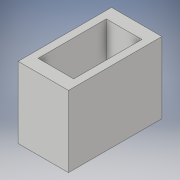
# Autodesk Inventor part: COXA_B
Saved by Autodesk Inventor 2017 (Build 210142000, 142)
## iProperties
Created: 2017-09-18
Part Number: COXA_B
Material: Generic
Document SubType Name: Modeling
Designer: Alexander Miller
Density: 1 g/cm^3
Appearance: Default
Author: Alexander Miller
Autodesk Inventor part; units mm, degrees
ref_plane "YZ Plane" through (0, 0, 0) normal (1, 0, 0) x (0, 1, 0)
ref_plane "XZ Plane" through (0, 0, 0) normal (0, 1, 0) x (-1, 0, 0)
ref_plane "XY Plane" through (0, 0, 0) normal (0, 0, 1) x (1, 0, 0)
sketch "Sketch1" plane through (0, 0, 0) normal (0, 1, 0) x (-1, 0, 0)
  line L0 (8.5, 15.75) -> (-8.5, 15.75)
  line L1 (-8.5, 15.75) -> (-8.5, -15.75)
  line L2 (-8.5, -15.75) -> (8.5, -15.75)
  line L3 (8.5, -15.75) -> (8.5, 15.75)
  point P0 (0, 0)
  point P1 (0, -15.75)
  point P2 (8.5, 0)
  dimension "d0" = 17
  dimension "d1" = 31.5
  constraints: 8 end point, 2 midpoint, 2 parallel, 1 horizontal, 1 horizontal alignment, 1 perpendicular, 1 vertical alignment
  measures "d0" distance of L1.end L2.end
  measures "d1" distance of L2.end L0.start
extrude "Extrusion1" add sketch "Sketch1" along normal blind 24
sketch "Sketch2" plane through (0, 24, 0) normal (0, 1, 0) x (1, 0, 0)
  line L0 (-6, -11.5) -> (6, -11.5)
  line L1 (6, -11.5) -> (6, 11.5)
  line L2 (6, 11.5) -> (-6, 11.5)
  line L3 (-6, 11.5) -> (-6, -11.5)
  point P0 (0, 0)
  point P1 (0, 11.5)
  point P2 (-6, 0)
  dimension "d4" = 12
  dimension "d5" = 23
  constraints: 8 end point, 2 midpoint, 2 parallel, 1 horizontal, 1 horizontal alignment, 1 perpendicular, 1 vertical alignment
  measures "d4" distance of L1.end L2.end
  measures "d5" distance of L2.end L0.start
extrude "Extrusion2" cut sketch "Sketch2" against normal blind 21
equation "\"d1\" = servo_D"
equation "\"d4\" = servo_B"
equation "\"d5\" = servo_A"
equation "\"d6\" = servo_E"
equation "\"servo_D\" = 31.5"
equation "\"servo_B\" = 12"
equation "\"servo_A\" = 23"
equation "\"servo_E\" = 21"
body "Solid1"
